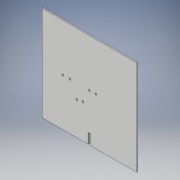
# Autodesk Inventor part: fs_roughmask
Saved by Autodesk Inventor 2017 (Build 210142000, 142)
## iProperties
Created: 2016-12-03
Part Number: fs_roughmask
Material: Generic
Document SubType Name: Modeling
Designer: Darien Morrow
Density: 1 g/cm^3
Appearance: Default
Author: Darien Morrow
Autodesk Inventor part; units mm, degrees
ref_plane "YZ Plane" through (0, 0, 0) normal (1, 0, 0) x (0, 1, 0)
ref_plane "XZ Plane" through (0, 0, 0) normal (0, 1, 0) x (-1, 0, 0)
ref_plane "XY Plane" through (0, 0, 0) normal (0, 0, 1) x (1, 0, 0)
sketch "Sketch1" plane through (0, 0, 0) normal (0, 0, 1) x (1, 0, 0)
  line L0 (-63.5, -63.5) -> (63.5, -63.5)
  line L1 (63.5, -63.5) -> (63.5, 63.5)
  line L2 (63.5, 63.5) -> (-63.5, 63.5)
  line L3 (-63.5, 63.5) -> (-63.5, -63.5)
  line L4 (-63.5, -63.5) -> (63.5, 63.5) construction
  line L5 (63.5, -63.5) -> (-63.5, 63.5) construction
  point P0 (0, 0)
  dimension "d0" = 127
  dimension "d1" = 127
  constraints: 12 end point, 2 midpoint, 2 parallel, 1 horizontal, 1 perpendicular
  measures "d0" distance between parallel lines of L1 L3
  measures "d1" distance between parallel lines of L0 L2
extrude "Extrusion1" add sketch "Sketch1" along normal blind 1.5875
sketch "Sketch2" plane through (0, 0, 0) normal (0, 0, -1) x (-1, 0, 0)
  line L0 (0, -76.2) -> (0, -50.8) construction
  line L1 (63.5, -63.5) -> (-63.5, -63.5) projected
  line L2 (1.5875, -76.2) -> (1.5875, -50.8)
  line L3 (-1.5875, -50.8) -> (-1.5875, -76.2)
  arc A0 (-1.5875, -76.2) -> (1.5875, -76.2) centre (0, -76.2) ccw
  arc A1 (1.5875, -50.8) -> (-1.5875, -50.8) centre (0, -50.8) ccw
  point P0 (0, 0)
  point P1 (0, -63.5)
  dimension "d4" = 12.7
  dimension "d5" = 3.175
  constraints: 8 end point, 4 point on circle, 4 tangent, 2 centre point, 2 midpoint, 1 parallel, 1 vertical
  measures "d4" distance of point (0, -63.5) L0.end
  measures "d5" diameter of A1
extrude "Extrusion2" cut sketch "Sketch2" against normal blind 1.5875
sketch "Sketch3" plane through (0, 0, 1.5875) normal (0, 0, 1) x (1, 0, 0)
  line L0 (-35.7187, 0) -> (2.3813, 0)
  line L1 (-16.6687, 0) -> (-16.6687, -19.05)
  line L2 (-63.5, 63.5) -> (-63.5, -63.5) projected
  line L3 (-26.1937, 0) -> (8.7313, 0)
  line L4 (-8.7312, 0) -> (-8.7312, -17.4625)
  point P0 (0, 0)
  point P1 (0, 0)
  dimension "d8" = 38.1
  dimension "d9" = 19.05
  dimension "d10" = 19.05
  dimension "d11" = 27.7812
  dimension "d12" = 34.925
  dimension "d13" = 9.525
  dimension "d14" = 17.4625
  dimension "d15" = 17.4625
  constraints: 8 end point, 6 coincident, 2 midpoint, 2 perpendicular, 2 point on line, 1 horizontal
  measures "d8" distance of L0.start L0.end
  measures "d9" distance of L1.start L1.end
  measures "d10" distance from line of L1 L0.start
  measures "d11" distance from line of L0.start L2
  measures "d12" distance of L3.start L3.end
  measures "d13" distance of L0.start L3.start
  measures "d14" distance of L4.start L4.end
  measures "d15" distance from line of L3.end L4
hole "Hole1" at (-35.7187, 0, 1.5875) at (-16.6687, -19.05, 1.5875) at (-26.1937, 0, 1.5875) at (-8.7312, -17.4625, 1.5875) at (8.7313, 0, 1.5875) at (0, 0, 1.5875) direction (0, 0, -1) diameter 2.54 depth 25.4 tip angle 118
body "Solid1"
